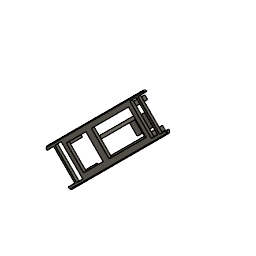
Titan_Dash_Panel_1 (Test 1.5) (Autodesk Fusion 360 design; units mm, degrees)
part number: 2026-08-09-09-25-20-493
Autodesk Fusion 360 part; units mm, degrees
sketch "Sketch1" plane through (0, 0, 0) normal (0, 0, 1) x (1, 0, 0)
  line L0 (134.62, 34.29) -> (-134.62, 34.29)
  line L1 (-134.62, 34.29) -> (-134.62, -34.29)
  line L2 (-134.62, -34.29) -> (134.62, -34.29)
  line L3 (134.62, -34.29) -> (134.62, 34.29)
  line L4 (134.62, 34.29) -> (-134.62, -34.29) construction
  line L5 (-134.62, 34.29) -> (134.62, -34.29) construction
  dimension "d8" = 269.24
  dimension "d9" = 68.58
  constraint horizontal L0
  constraint perpendicular L0 L1
  constraint parallel L0 L2
  constraint parallel L1 L3
  constraint coincident L4 origin
  constraint coincident L5 origin
  measures "d8" distance of L1.end L2.end
  measures "d9" distance of L0.end L1.end
extrude "Extrude1" add sketch "Sketch1" along normal blind 5.08
fillet "Fillet1" [suppressed]
sketch "Sketch2" plane through (0, 0, 0) normal (0, 0, -1) x (-1, 0, 0)
  line L0 (-134.62, 34.29) -> (-134.62, -34.29)
  line L1 (-134.62, -34.29) -> (134.62, -34.29)
  line L2 (134.62, -34.29) -> (134.62, 34.29)
  line L3 (134.62, 34.29) -> (-134.62, 34.29)
  line L4 (90.17, -27.94) -> (-90.17, -27.94)
  line L5 (-90.17, -27.94) -> (-90.17, 27.94)
  line L6 (-90.17, 27.94) -> (90.17, 27.94)
  line L7 (90.17, 27.94) -> (90.17, -27.94)
  line L8 (90.17, -27.94) -> (-90.17, 27.94) construction
  line L9 (-90.17, -27.94) -> (90.17, 27.94) construction
  line L10 (21.9978, -27.94) -> (27.0778, -27.94)
  line L11 (27.0778, -27.94) -> (27.0778, 22.86)
  line L12 (27.0778, 22.86) -> (21.9978, 22.86)
  line L13 (21.9978, 22.86) -> (21.9978, -27.94)
  dimension "d14" = 180.34
  dimension "d15" = 55.88
  dimension "d39" = 5.08
  constraint horizontal L4
  constraint perpendicular L4 L5
  constraint parallel L4 L6
  constraint parallel L5 L7
  constraint coincident L8 origin
  constraint coincident L9 origin
  constraint horizontal L10
  constraint vertical L11
  constraint horizontal L12
  constraint vertical L13
  constraint coincident L4 L10.start
  measures "d14" distance of L5.end L6.end
  measures "d15" distance of L4.end L5.end
  measures "d39" distance of L10.start L10.end
sketch "Sketch3" plane through (0, 0, 0) normal (0, 0, -1) x (-1, 0, 0)
sketch "Sketch4" plane through (0, 0, 0) normal (0, 0, -1) x (-1, 0, 0)
  line L0 (-90.17, 27.94) -> (90.17, 27.94)
  line L1 (-90.17, -27.94) -> (-90.17, 27.94)
  line L2 (90.17, -27.94) -> (-90.17, -27.94)
  line L3 (90.17, 27.94) -> (90.17, -27.94)
  line L4 (-90.17, 27.94) -> (-82.55, 27.94)
  line L5 (-82.55, 27.94) -> (-82.55, 25.4)
  line L6 (-82.55, 25.4) -> (-90.17, 25.4)
  line L7 (-90.17, 25.4) -> (-90.17, 27.94)
  line L8 (-90.17, 27.94) -> (-87.63, 27.94)
  line L9 (-87.63, 27.94) -> (-87.63, 20.32)
  line L10 (-87.63, 20.32) -> (-90.17, 20.32)
  line L11 (-90.17, 20.32) -> (-90.17, 27.94)
  line L12 (-90.17, -27.94) -> (-87.63, -27.94)
  line L13 (-87.63, -27.94) -> (-87.63, -20.32)
  line L14 (-87.63, -20.32) -> (-90.17, -20.32)
  line L15 (-90.17, -20.32) -> (-90.17, -27.94)
  line L16 (-90.17, -27.94) -> (-87.63, -27.94)
  line L17 (-87.63, -27.94) -> (-87.63, -20.32)
  line L18 (-87.63, -20.32) -> (-90.17, -20.32)
  line L19 (-90.17, -20.32) -> (-90.17, -27.94)
  line L20 (-90.17, -27.94) -> (-82.55, -27.94)
  line L21 (-82.55, -27.94) -> (-82.55, -25.4)
  line L22 (-82.55, -25.4) -> (-90.17, -25.4)
  line L23 (-90.17, -25.4) -> (-90.17, -27.94)
  line L24 (90.17, 27.94) -> (82.55, 27.94)
  line L25 (82.55, 27.94) -> (82.55, 25.4)
  line L26 (82.55, 25.4) -> (90.17, 25.4)
  line L27 (90.17, 25.4) -> (90.17, 27.94)
  line L28 (90.17, 27.94) -> (87.63, 27.94)
  line L29 (87.63, 27.94) -> (87.63, 20.32)
  line L30 (87.63, 20.32) -> (90.17, 20.32)
  line L31 (90.17, 20.32) -> (90.17, 27.94)
  line L32 (90.17, -27.94) -> (87.63, -27.94)
  line L33 (87.63, -27.94) -> (87.63, -20.32)
  line L34 (87.63, -20.32) -> (90.17, -20.32)
  line L35 (90.17, -20.32) -> (90.17, -27.94)
  line L36 (90.17, -27.94) -> (82.55, -27.94)
  line L37 (82.55, -27.94) -> (82.55, -25.4)
  line L38 (82.55, -25.4) -> (90.17, -25.4)
  line L39 (90.17, -25.4) -> (90.17, -27.94)
  dimension "d17" = 7.62
  dimension "d18" = 2.54
  dimension "d19" = 2.54
  dimension "d20" = 7.62
  dimension "d21" = 2.54
  dimension "d22" = 7.62
  dimension "d23" = 2.54
  dimension "d24" = 7.62
  dimension "d25" = 7.62
  dimension "d26" = 2.54
  dimension "d27" = 7.62
  dimension "d28" = 2.54
  dimension "d29" = 2.54
  dimension "d30" = 7.62
  dimension "d31" = 2.54
  dimension "d32" = 7.62
  dimension "d33" = 7.62
  dimension "d34" = 2.54
  constraint horizontal L4
  constraint vertical L5
  constraint horizontal L6
  constraint vertical L7
  constraint coincident L0.start L1.end
  constraint horizontal L8
  constraint vertical L9
  constraint horizontal L10
  constraint vertical L11
  constraint horizontal L12
  constraint vertical L13
  constraint horizontal L14
  constraint vertical L15
  constraint coincident L1.start L2.end
  constraint horizontal L16
  constraint vertical L17
  constraint horizontal L18
  constraint vertical L19
  constraint horizontal L20
  constraint vertical L21
  constraint horizontal L22
  constraint vertical L23
  constraint horizontal L24
  constraint vertical L25
  constraint horizontal L26
  constraint vertical L27
  constraint coincident L0.end L3.start
  constraint horizontal L28
  constraint vertical L29
  constraint horizontal L30
  constraint vertical L31
  constraint horizontal L32
  constraint vertical L33
  constraint horizontal L34
  constraint vertical L35
  constraint coincident L2.start L3.end
  constraint horizontal L36
  constraint vertical L37
  constraint horizontal L38
  constraint vertical L39
  measures "d17" distance of L0.start L4.end
  measures "d18" distance of L0.start L6.end
  measures "d19" distance of L0.start L8.end
  measures "d20" distance of L0.start L10.end
  measures "d21" distance of L1.start L12.end
  measures "d22" distance of L1.start L14.end
  measures "d23" distance of L1.start L12.end
  measures "d24" distance of L1.start L14.end
  measures "d25" distance of L1.start L20.end
  measures "d26" distance of L1.start L22.end
  measures "d27" distance of L0.end L24.end
  measures "d28" distance of L0.end L26.end
  measures "d29" distance of L0.end L28.end
  measures "d30" distance of L0.end L30.end
  measures "d31" distance of L2.start L32.end
  measures "d32" distance of L2.start L34.end
  measures "d33" distance of L2.start L36.end
  measures "d34" distance of L2.start L38.end
extrude "Extrude2" add sketch "Sketch4" along normal blind 25.4 contours L0 L1 L4 L6 L7 L8 L9 L11 | L0 L4 L5 L6 L9 | L1 L6 L9 L10 L11 | L0 L24 L25 L26 L29 | L1 L13 L14 L15 L17 L18 L19 L22 | L0 L3 L24 L26 L27 L28 L29 L31 | L1 L2 L12 L13 L15 L16 L17 L19 L20 L22 L23 | L3 L26 L29 L30 L31 | L2 L13 L17 L20 L21 L22 | L3 L33 L34 L35 L38 | L2 L33 L36 L37 L38 | L2 L3 L32 L33 L35 L36 L38 L39
extrude "Extrude4" add sketch "Sketch2" along normal blind 76.2 contours L4 L10 L11 L12 L13
sketch "Sketch5" plane through (0, 0, -76.2) normal (0, 0, -1) x (-1, 0, 0)
  line L0 (21.9978, 22.86) -> (21.9978, -27.94)
  line L1 (21.9978, -27.94) -> (27.0778, -27.94)
  line L2 (27.0778, -27.94) -> (27.0778, 22.86)
  line L3 (27.0778, 22.86) -> (21.9978, 22.86)
  line L4 (46.5284, -16.0632) -> (2.1272, -16.0632)
  line L5 (2.1272, -16.0632) -> (2.1272, 6.9831)
  line L6 (2.1272, 6.9831) -> (46.5284, 6.9831)
  line L7 (46.5284, 6.9831) -> (46.5284, -16.0632)
  line L8 (46.5284, -16.0632) -> (2.1272, 6.9831) construction
  line L9 (2.1272, -16.0632) -> (46.5284, 6.9831) construction
  point P0 (24.3278, -4.54)
  constraint horizontal L4
  constraint perpendicular L4 L5
  constraint parallel L4 L6
  constraint parallel L5 L7
  constraint coincident L8 P0
  constraint coincident L9 P0
extrude "Extrude5" add sketch "Sketch5" along normal blind 2.54 contours L0 L2 L4 L6 | L0 L4 L5 L6 | L2 L4 L6 L7
sketch "Sketch6" plane through (0, 0, 5.08) normal (0, 0, 1) x (1, 0, 0)
  line L0 (-27.0778, -27.94) -> (-27.0778, 22.86)
  line L1 (-21.9978, 22.86) -> (-21.9978, -27.94)
  line L2 (-84.4681, 24.2382) -> (-31.4836, 24.2382)
  line L3 (-31.4836, 24.2382) -> (-31.4836, -22.6712)
  line L4 (-31.4836, -22.6712) -> (-84.4681, -22.6712)
  line L5 (-84.4681, -22.6712) -> (-84.4681, 24.2382)
  line L6 (-15.8698, 24.4915) -> (84.98, 24.4915)
  line L7 (84.98, 24.4915) -> (84.98, -23.4013)
  line L8 (84.98, -23.4013) -> (-15.8698, -23.4013)
  line L9 (-15.8698, -23.4013) -> (-15.8698, 24.4915)
  line L10 (111.9771, 30.423) -> (95.1039, 30.423)
  line L11 (95.1039, 30.423) -> (95.1039, -28.1221)
  line L12 (95.1039, -28.1221) -> (111.9771, -28.1221)
  line L13 (111.9771, -28.1221) -> (111.9771, 30.423)
  line L14 (-93.8256, 29.4004) -> (-110.6989, 29.4004)
  line L15 (-110.6989, 29.4004) -> (-110.6989, -29.4004)
  line L16 (-110.6989, -29.4004) -> (-93.8256, -29.4004)
  line L17 (-93.8256, -29.4004) -> (-93.8256, 29.4004)
  line L18 (134.62, -34.29) -> (134.62, 34.29)
  line L19 (134.62, 34.29) -> (-134.62, 34.29)
  line L20 (-134.62, 34.29) -> (-134.62, -34.29)
  line L21 (-134.62, -34.29) -> (134.62, -34.29)
  line L22 (-135.0248, 28.8288) -> (-115.0211, 28.8288)
  line L23 (-115.0211, 28.8288) -> (-115.0211, -28.8288)
  line L24 (-115.0211, -28.8288) -> (-135.0248, -28.8288)
  line L25 (-135.0248, -28.8288) -> (-135.0248, 28.8288)
  line L26 (116.7861, 30.423) -> (134.7306, 30.423)
  line L27 (134.7306, 30.423) -> (134.7306, -28.8288)
  line L28 (134.7306, -28.8288) -> (116.7861, -28.8288)
  line L29 (116.7861, -28.8288) -> (116.7861, 30.423)
  constraint horizontal L2
  constraint vertical L3
  constraint horizontal L4
  constraint vertical L5
  constraint horizontal L6
  constraint vertical L7
  constraint horizontal L8
  constraint vertical L9
  constraint horizontal L10
  constraint vertical L11
  constraint horizontal L12
  constraint vertical L13
  constraint horizontal L14
  constraint vertical L15
  constraint horizontal L16
  constraint vertical L17
  constraint horizontal L22
  constraint vertical L23
  constraint horizontal L24
  constraint vertical L25
  constraint horizontal L26
  constraint vertical L27
  constraint horizontal L28
  constraint vertical L29
extrude "Extrude6" cut sketch "Sketch6" against normal blind 12.7 contours L2 L3 L4 L5 | L6 L7 L8 L9 | L10 L11 L12 L13 | L14 L15 L16 L17 | L18 L26 L28 L29 | L18 L26 L27 L28 | L20 L22 L24 L25 | L20 L22 L23 L24
fillet "Fillet3" radius 5.08 4 edges at (134.62, 34.29, 2.54) (134.62, -34.29, 2.54) (-134.62, 34.29, 2.54) (-134.62, -34.29, 2.54)
fillet "Fillet4" radius 1.27 9 edges at (0.0735, 34.29, 5.08) (132.821, 33.208, 5.08) (134.62, -29.0194, 5.08) (133.1321, -32.8021, 5.08) (0, -34.29, 5.08) (-133.1321, -32.8021, 5.08) (-134.62, -29.0194, 5.08) (-134.62, 29.0194, 5.08) (-133.1321, 32.8021, 5.08)
move_body "Move1" bodies 1 to x (0.707107, 0.707107, 0) y (-0.707107, 0.707107, 0) z (0, 0, 1) at (-3.8333, 0.1744, 0)
sketch "Sketch9" plane through (-17.3843, -17.3843, 0) normal (0.707107, 0.707107, 0) x (0, 0, -1)
  line L0 (0, 25.6939) -> (0, -25.1061)
  line L1 (0, -25.1061) -> (76.2, -25.1061)
  line L2 (76.2, -25.1061) -> (76.2, -13.2293)
  line L3 (76.2, -13.2293) -> (76.2, 9.817)
  line L4 (76.2, 9.817) -> (76.2, 25.6939)
  line L5 (76.2, 25.6939) -> (0, 25.6939)
  line L6 (76.2, 13.3999) -> (0, 13.3999)
  line L7 (0, 13.3999) -> (0, 25.6939)
  line L8 (0, 25.6939) -> (76.2, 25.6939)
  line L9 (76.2, 25.6939) -> (76.2, 13.3999)
  constraint horizontal L6
  constraint vertical L7
  constraint horizontal L8
  constraint vertical L9
  constraint coincident L0.start L5.end
  constraint coincident L4 L6.start
extrude "Extrude8" cut sketch "Sketch9" against normal blind 5.08 contours L0 L4 L5 L6 L7 L8 L9
sketch "Sketch10" plane through (-17.3843, -17.3843, 0) normal (0.707107, 0.707107, 0) x (0, 0, -1)
  line L0 (76.2, 13.3999) -> (0, 13.3999)
  line L1 (0, 13.3999) -> (0, -25.1061)
  line L2 (0, -25.1061) -> (76.2, -25.1061)
  line L3 (76.2, -25.1061) -> (76.2, -13.2293)
  line L4 (76.2, -13.2293) -> (76.2, 9.817)
  line L5 (76.2, 9.817) -> (76.2, 13.3999)
  line L6 (4.2884, 8.0408) -> (72.903, 8.0408)
  line L7 (72.903, 8.0408) -> (72.903, -17.9577)
  line L8 (72.903, -17.9577) -> (4.2884, -17.9577)
  line L9 (4.2884, -17.9577) -> (4.2884, 8.0408)
  constraint horizontal L6
  constraint vertical L7
  constraint horizontal L8
  constraint vertical L9
extrude "Extrude9" cut sketch "Sketch10" against normal blind 5.08 contours L6 L7 L8 L9
fillet "Fillet5" radius 2.54 2 edges at (-16.8376, -25.1151, 0) (-13.2455, -21.523, 0)
fillet "Fillet6" radius 2.54 2 edges at (-19.7699, -22.1828, -76.2) (-13.8781, -20.8904, -72.903)
extrude "Extrude3" [suppressed]
equation "panelWidth = innerWidth + 2 * widthMargin"
equation "panelHeight = innerHeight + heightMargin"
equation "panelThickness = 0.2 in"
equation "panelFrontFillet = 0.1 in"
equation "bossThickness = 0.1 in"
equation "innerWidth = 7.1 in"
equation "innerHeight = 2.2 in"
equation "d8 = panelWidth"
equation "d9 = panelHeight"
equation "d10 = panelThickness"
equation "d13 = panelFrontFillet"
equation "d14 = innerWidth"
equation "d15 = innerHeight"
equation "bossWidth = 0.3 in"
equation "d17 = bossWidth"
equation "d18 = bossThickness"
equation "d19 = bossThickness"
equation "d20 = bossWidth"
equation "d21 = bossThickness"
equation "d22 = bossWidth"
equation "d23 = bossThickness"
equation "d24 = bossWidth"
equation "d25 = bossWidth"
equation "d26 = bossThickness"
equation "d27 = bossWidth"
equation "d28 = bossThickness"
equation "d29 = bossThickness"
equation "d30 = bossWidth"
equation "d31 = bossThickness"
equation "d32 = bossWidth"
equation "d33 = bossWidth"
equation "d34 = bossThickness"
equation "widthMargin = 1.75 in"
equation "heightMargin = 0.5 in"
